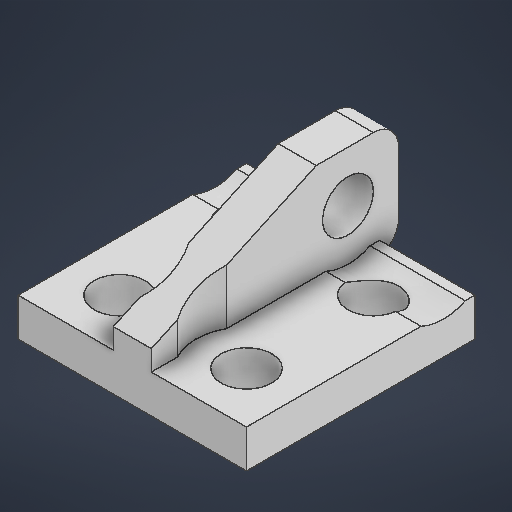
# Autodesk Inventor part: link2
Saved by Autodesk Inventor 2026.1 (Build 301233000, 233)
## iProperties
Created: 2026-05-13
Part Number: link2
Material: Generic
Document SubType Name: Modeling
Designer: emanuel
Density: 1 g/cm^3
Appearance: Default
Author: emanuel
Autodesk Inventor part; units mm, degrees
ref_plane "YZ Plane" through (0, 0, 0) normal (1, 0, 0) x (0, 1, 0)
ref_plane "XZ Plane" through (0, 0, 0) normal (0, 1, 0) x (-1, 0, 0)
ref_plane "XY Plane" through (0, 0, 0) normal (0, 0, 1) x (1, 0, 0)
sketch "Sketch1" plane through (0, 0, 0) normal (0, 1, 0) x (-1, 0, 0)
  line L0 (-5, 5) -> (5, 5)
  line L1 (5, 5) -> (5, -5)
  line L2 (5, -5) -> (-5, -5)
  line L3 (-5, -5) -> (-5, 5)
  line L4 (-5, 5) -> (5, -5) construction
  line L5 (5, 5) -> (-5, -5) construction
  line L6 (-9, 9) -> (9, 9)
  line L7 (9, 9) -> (9, -9)
  line L8 (9, -9) -> (-9, -9)
  line L9 (-9, -9) -> (-9, 9)
  line L10 (-9, 9) -> (9, -9) construction
  line L11 (9, 9) -> (-9, -9) construction
  circle A0 centre (5, 5) radius 2
  circle A1 centre (-5, 5) radius 2
  circle A2 centre (5, -5) radius 2
  circle A3 centre (-5, -5) radius 2
  point P0 (0, 0)
  dimension "d0" = 10
  dimension "d1" = 10
  dimension "d2" = 18
  dimension "d3" = 18
  dimension "d4" = 4
  dimension "d5" = 4
  dimension "d6" = 4
  dimension "d7" = 4
  constraints: 24 end point, 4 centre point, 4 coincident, 4 midpoint, 4 parallel, 2 horizontal, 2 perpendicular
  measures "d0" distance of L1.end L2.end
  measures "d1" distance of L0.end L1.end
  measures "d2" distance of L7.end L8.end
  measures "d3" distance of L6.end L7.end
  measures "d4" diameter of A0
  measures "d5" diameter of A1
  measures "d6" diameter of A2
  measures "d7" diameter of A3
extrude "Extrusion1" add sketch "Sketch1" along normal blind 3 contours L0 A0 L1 A2 L2 A3 L3 A1 | L6 L7 L8 L9
sketch "Sketch2" plane through (0, 3, 0) normal (0, 1, 0) x (1, 0, 0)
  line L0 (9, 9) -> (-9, 9) projected
  line L1 (1.5, -9) -> (-1.5, -9)
  line L2 (-1.5, -9) -> (-1.5, 9)
  line L3 (-1.5, 9) -> (1.5, 9)
  line L4 (1.5, 9) -> (1.5, -9)
  line L5 (1.5, -9) -> (-1.5, 9) construction
  line L6 (-1.5, -9) -> (1.5, 9) construction
  circle A0 centre (-5, -5) radius 2 projected
  circle A1 centre (-5, -5) radius 4
  circle A2 centre (-5, 5) radius 2 projected
  circle A3 centre (-5, 5) radius 4
  circle A4 centre (5, -5) radius 2 projected
  circle A5 centre (5, -5) radius 4
  circle A6 centre (5, 5) radius 2 projected
  circle A7 centre (5, 5) radius 4
  point P0 (0, 0)
  point P1 (1.5, -6.9365)
  point P2 (1.5, -3.0635)
  point P3 (1.5, 3.0635)
  point P4 (1.5, 6.9365)
  point P5 (-1.5, 6.9365)
  point P6 (-1.5, 3.0635)
  point P7 (-1.5, -3.0635)
  point P8 (-1.5, -6.9365)
  dimension "d10" = 3
  dimension "d11" = 8
  dimension "d12" = 8
  dimension "d13" = 8
  dimension "d14" = 8
  constraints: 12 end point, 4 centre point, 4 coincident, 2 midpoint, 2 parallel, 1 horizontal, 1 perpendicular, 1 point on line
  measures "d10" distance of L2.end L3.end
  measures "d11" diameter of A1
  measures "d12" diameter of A3
  measures "d13" diameter of A5
  measures "d14" diameter of A7
extrude "Extrusion2" add sketch "Sketch2" along normal blind 7.6 contours L4 A7 A5 L1 L2 A1 A3 L0
sketch "Sketch3" plane through (1.5, 3, 9) normal (1, 0, 0) x (0, 0, -1)
  line L0 (0, -3) -> (0, 0) projected
  line L1 (0, -3) -> (0, 3.6)
  line L2 (0, 3.6) -> (18, 3.6)
  line L3 (18, 0) -> (18, 7.6) projected
  line L4 (18, 3.6) -> (15.5, 3.6)
  circle A0 centre (15.5, 3.6) radius 2
  circle A1 centre (15.5, 3.6) radius 4
  line L5 (19.5, -0.4) -> (11.5, -0.4)
  line L6 (11.5, -0.4) -> (11.5, 7.6)
  line L7 (11.5, 7.6) -> (19.5, 7.6)
  line L8 (19.5, 7.6) -> (19.5, -0.4)
  line L9 (19.5, -0.4) -> (11.5, 7.6) construction
  line L10 (11.5, -0.4) -> (19.5, 7.6) construction
  point P0 (9, -3)
  dimension "d17" = 6.6
  dimension "d18" = 2.5
  dimension "d19" = 4
  dimension "d20" = 8
  constraints: 18 end point, 2 centre point, 2 coincident, 2 midpoint, 2 parallel, 2 perpendicular, 2 point on line, 1 collinear, 1 horizontal
  measures "d17" distance of L0.start L1.end
  measures "d18" distance of L2.end L4.end
  measures "d19" diameter of A0
  measures "d20" diameter of A1
extrude "Extrusion3" add sketch "Sketch3" against normal up to surface (3 mm away)
extrude "Extrusion4" cut sketch "Sketch3" against normal blind 10 contours L2 A0 | L2 A0
extrude "Extrusion5" cut sketch "Sketch3" along normal blind 10 contours L2 A0 | L2 A0 | A0 L2 A1 L3 | L2 L3 A1 A0 | L3 A1
extrude "Extrusion6" cut sketch "Sketch3" against normal blind 20 contours L2 A0 | L2 A0 | A0 L2 A1 L3 | L2 L3 A1 A0 | L3 A1
extrude "Extrusion7" add sketch "Sketch3" against normal up to surface (3 mm away) contours A0 L2 A1 L3 | L2 L3 A1 A0 | L3 A1
chamfer "Chamfer1" distance 13 distance2 6 1 edges at (0, 10.6, 9) measured on face at (-0.5, 10.6, -5.9788)
fillet "Fillet1" radius 2 3 edges at (0, 10.6, -10.5) (0, 2.6, -10.5) (0, 2.6, -9)
body "Solid1"
